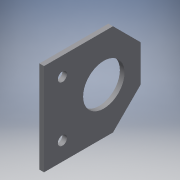
# Autodesk Inventor part: 15102898-16-P-0302
Saved by Autodesk Inventor 2017 (Build 210142000, 142)
## iProperties
Created: 2016-10-02
Part Number: 15102898-16-P-0302
Material: Aluminum 6061
Document SubType Name: Modeling
Designer: gus
Density: 2.7 g/cm^3
Appearance: Aluminum - Flat
Author: gus
Autodesk Inventor part; units mm, degrees
ref_plane "YZ Plane" through (0, 0, 0) normal (1, 0, 0) x (0, 1, 0)
ref_plane "XZ Plane" through (0, 0, 0) normal (0, 1, 0) x (-1, 0, 0)
ref_plane "XY Plane" through (0, 0, 0) normal (0, 0, 1) x (1, 0, 0)
sketch "Sketch1" plane through (0, 0, 0) normal (1, 0, 0) x (0, 1, 0)
  line L0 (0, 0) -> (63.5, 0)
  line L1 (63.5, 0) -> (63.5, -47.625)
  line L2 (63.5, -47.625) -> (44.45, -66.675)
  line L3 (44.45, -66.675) -> (19.05, -66.675)
  line L4 (19.05, -66.675) -> (0, -47.625)
  line L5 (0, -47.625) -> (0, 0)
  circle A0 centre (31.75, -41.275) radius 14.2875
  line L6 (63.5, -25.4) -> (0, -25.4) construction
  circle A1 centre (50.8, -12.7) radius 3.175
  circle A2 centre (12.7, -12.7) radius 3.175
  dimension "d0" = 47.625
  dimension "d1" = 28.575
  dimension "d2" = 63.5
  dimension "d3" = 19.05
  dimension "d4" = 25.4
  dimension "d5" = 31.75
  dimension "d6" = 25.4
  dimension "d7" = 6.35
  dimension "d8" = 6.35
  dimension "d9" = 12.7
  dimension "d10" = 12.7
  dimension "d11" = 12.7
  dimension "d12" = 12.7
  constraints: 14 end point, 3 centre point, 3 perpendicular, 2 equal length, 2 parallel, 2 point on line, 1 horizontal
  measures "d0" distance of L0.end L1.end
  measures "d1" diameter of A0
  measures "d2" distance of L0.start L0.end
  measures "d3" distance from line of L4.end L3
  measures "d4" distance from line of L3 A0.centre
  measures "d5" distance from line of L1 A0.centre
  measures "d6" distance between parallel lines of L0 L6
  measures "d7" diameter of A1
  measures "d8" diameter of A2
  measures "d9" distance from line of L6 A2.centre
  measures "d10" distance from line of L6 A1.centre
  measures "d11" distance from line of L5 A2.centre
  measures "d12" distance from line of L1 A1.centre
extrude "Extrusion1" add sketch "Sketch1" along normal blind 6.35
body "Solid1"
